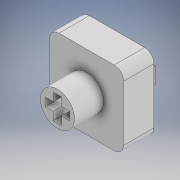
# Autodesk Inventor part: IPC MARK 7 key
Saved by Autodesk Inventor 2022 (Build 260153000, 153)
## iProperties
Created: 2021-12-31
Part Number: IPC MARK 7 key
Material: Generic
Document SubType Name: Modeling
Designer: solor
Density: 1 g/cm^3
Appearance: Default
Author: solor
Autodesk Inventor part; units mm, degrees
ref_plane "YZ Plane" through (0, 0, 0) normal (1, 0, 0) x (0, 1, 0)
ref_plane "XZ Plane" through (0, 0, 0) normal (0, 1, 0) x (-1, 0, 0)
sketch "Sketch1" plane through (0, 0, 0) normal (0, 0, 1) x (1, 0, 0)
  line L0 (14.6962, 12.74) -> (14.6962, 0) construction
  line L1 (10.61, 12.2) -> (1.53, 12.2)
  arc A0 (1.53, 12.2) -> (0, 10.67) centre (1.53, 10.67) ccw
  line L2 (0, 10.67) -> (0, 1.53)
  arc A1 (0, 1.53) -> (1.53, 0) centre (1.53, 1.53) ccw
  line L3 (1.53, 0) -> (10.61, 0)
  arc A2 (10.61, 0) -> (12.14, 1.53) centre (10.61, 1.53) ccw
  arc A3 (12.14, 10.67) -> (10.61, 12.2) centre (10.61, 10.67) ccw
  line L4 (12.14, 10.67) -> (12.14, 1.53)
  point P0 (0, 0)
  point P1 (0, 0)
  dimension "d10" = 12.74
  constraints: 10 end point, 8 point on circle, 4 centre point, 2 vertical, 1 point on line
  measures "d10" distance of L0.start L0.end
ref_plane "Work Plane1" through (0, 0, 5) normal (0, 0, 1) x (1, 0, 0)
sketch "Sketch2" plane through (0, 0, 5) normal (0, 0, 1) x (1, 0, 0)
  line L0 (10.88, 12.74) -> (1.8, 12.74) projected
  line L1 (10.88, 12.74) -> (1.8, 12.74) projected
  arc A0 (1.8, 12.74) -> (0, 10.94) centre (1.8, 10.94) ccw projected
  line L2 (0, 10.94) -> (0, 1.8) projected
  arc A1 (0, 1.8) -> (1.8, 0) centre (1.8, 1.8) ccw projected
  line L3 (1.8, 0) -> (10.88, 0) projected
  arc A2 (10.88, 0) -> (12.68, 1.8) centre (10.88, 1.8) ccw projected
  line L4 (12.68, 1.8) -> (12.68, 10.94) projected
  arc A3 (12.68, 10.94) -> (10.88, 12.74) centre (10.88, 10.94) ccw projected
  circle A4 centre (6.34, 6.37) radius 2.8
  line L5 (5.665, 8.395) -> (7.015, 8.395)
  line L6 (7.015, 4.345) -> (5.665, 4.345)
  line L7 (5.665, 4.345) -> (7.015, 8.395) construction
  line L8 (5.665, 8.395) -> (7.015, 4.345) construction
  line L9 (8.365, 5.695) -> (8.365, 7.045)
  line L10 (4.315, 7.045) -> (4.315, 5.695)
  line L11 (4.315, 5.695) -> (8.365, 7.045) construction
  line L12 (8.365, 5.695) -> (4.315, 7.045) construction
  line L13 (4.315, 5.695) -> (5.665, 5.695)
  line L14 (7.015, 5.695) -> (8.365, 5.695)
  line L15 (5.665, 4.345) -> (5.665, 5.695)
  line L16 (5.665, 7.045) -> (5.665, 8.395)
  line L17 (8.365, 7.045) -> (7.015, 7.045)
  line L18 (5.665, 7.045) -> (4.315, 7.045)
  line L19 (7.015, 8.395) -> (7.015, 7.045)
  line L20 (7.015, 5.695) -> (7.015, 4.345)
  point P0 (0, 0)
  dimension "d3" = 5.6
  dimension "d4" = 4.05
  dimension "d5" = 1.35
  dimension "d6" = 4.05
  dimension "d7" = 1.35
  constraints: 32 end point, 10 parallel, 8 perpendicular, 4 midpoint, 2 vertical, 1 centre point
  measures "d3" diameter of A4
  measures "d4" distance of L6.end L5.start
  measures "d5" distance of L5.start L5.end
  measures "d6" distance of L10.end L9.start
  measures "d7" distance of L9.end L9.start
extrude "Extrusion3" add sketch "Sketch1" along normal blind 5
sketch "Sketch3" plane through (0, 0, 5) normal (0, 0, 1) x (1, 0, 0)
  line L0 (10.61, 12.47) -> (1.53, 12.47)
  line L1 (10.61, 12.47) -> (1.53, 12.47)
  arc A0 (1.53, 12.47) -> (-0.27, 10.67) centre (1.53, 10.67) ccw
  line L2 (-0.27, 10.67) -> (-0.27, 1.53)
  arc A1 (-0.27, 1.53) -> (1.53, -0.27) centre (1.53, 1.53) ccw
  line L3 (1.53, -0.27) -> (10.61, -0.27)
  arc A2 (10.61, -0.27) -> (12.41, 1.53) centre (10.61, 1.53) ccw
  line L4 (12.41, 1.53) -> (12.41, 10.67)
  arc A3 (12.41, 10.67) -> (10.61, 12.47) centre (10.61, 10.67) ccw
  circle A4 centre (6.07, 6.1) radius 2.8
  line L5 (5.395, 8.125) -> (6.745, 8.125)
  line L6 (6.745, 4.075) -> (5.395, 4.075)
  line L7 (5.395, 4.075) -> (6.745, 8.125) construction
  line L8 (5.395, 8.125) -> (6.745, 4.075) construction
  line L9 (8.095, 5.425) -> (8.095, 6.775)
  line L10 (4.045, 6.775) -> (4.045, 5.425)
  line L11 (4.045, 5.425) -> (8.095, 6.775) construction
  line L12 (8.095, 5.425) -> (4.045, 6.775) construction
  line L13 (4.045, 5.425) -> (5.395, 5.425)
  line L14 (6.745, 5.425) -> (8.095, 5.425)
  line L15 (5.395, 4.075) -> (5.395, 5.425)
  line L16 (5.395, 6.775) -> (5.395, 8.125)
  line L17 (8.095, 6.775) -> (6.745, 6.775)
  line L18 (5.395, 6.775) -> (4.045, 6.775)
  line L19 (6.745, 8.125) -> (6.745, 6.775)
  line L20 (6.745, 5.425) -> (6.745, 4.075)
  line L21 (10.61, 12.2) -> (1.53, 12.2) projected
  line L22 (0, 10.67) -> (0, 1.53) projected
  point P0 (0, 0)
  point P1 (-0.27, -0.27)
  point P2 (6.07, 12.2)
  point P3 (0, 6.1)
  point P4 (6.07, 6.1)
  dimension "d14" = 5.6
  dimension "d15" = 4.05
  dimension "d16" = 1.35
  dimension "d17" = 4.05
  dimension "d18" = 1.35
  constraints: 42 end point, 10 parallel, 8 perpendicular, 8 point on circle, 6 midpoint, 5 centre point, 2 vertical
  measures "d14" diameter of A4
  measures "d15" distance of L6.end L5.start
  measures "d16" distance of L5.start L5.end
  measures "d17" distance of L10.end L9.start
  measures "d18" distance of L9.end L9.start
extrude "Extrusion4" add sketch "Sketch3" along normal blind 4.8 contours A4
sketch "Sketch4" plane through (0, 0, 0) normal (0, 0, -1) x (-1, 0, 0)
  line L0 (-13.9436, 0) -> (-13.9436, 2.266)
  line L1 (-15.5559, 0) -> (-15.5559, 6.84)
  line L2 (-1.53, 0) -> (-10.61, 0) projected
  line L3 (-11.7556, 9.6007) -> (-0.3844, 9.6007) construction
  line L4 (-0.3844, 9.6007) -> (-0.3844, 6.84) construction
  line L5 (-0.3844, 6.84) -> (-11.7556, 6.84) construction
  line L6 (-11.7556, 6.84) -> (-11.7556, 9.6007) construction
  line L7 (-7.4059, 5.316) -> (-4.7341, 5.316) construction
  line L8 (-4.7341, 5.316) -> (-4.7341, 2.266) construction
  line L9 (-4.7341, 2.266) -> (-7.4059, 2.266) construction
  line L10 (-7.4059, 2.266) -> (-7.4059, 5.316) construction
  line L11 (-8.7186, 6.9007) -> (-9.3925, 6.9007)
  line L12 (-9.3925, 6.9007) -> (-9.3925, 8.6905)
  line L13 (-9.3925, 8.6905) -> (-9.8826, 7.5352)
  line L14 (-9.8826, 7.5352) -> (-10.3465, 7.5352)
  line L15 (-10.3465, 7.5352) -> (-10.8366, 8.6905)
  line L16 (-10.8366, 8.6905) -> (-10.8366, 6.9007)
  line L17 (-10.8366, 6.9007) -> (-11.4755, 6.9007)
  line L18 (-11.4755, 6.9007) -> (-11.4755, 9.6007)
  line L19 (-11.4755, 9.6007) -> (-10.6944, 9.6007)
  line L20 (-10.6944, 9.6007) -> (-10.0949, 8.2682)
  line L21 (-10.0949, 8.2682) -> (-9.4997, 9.6007)
  line L22 (-9.4997, 9.6007) -> (-8.7186, 9.6007)
  line L23 (-8.7186, 9.6007) -> (-8.7186, 6.9007)
  line L24 (-8.4495, 6.9007) -> (-7.5371, 9.6007)
  line L25 (-7.5371, 9.6007) -> (-6.7976, 9.6007)
  line L26 (-6.7976, 9.6007) -> (-5.8852, 6.9007)
  line L27 (-5.8852, 6.9007) -> (-6.5831, 6.9007)
  line L28 (-6.5831, 6.9007) -> (-6.7516, 7.4521)
  line L29 (-6.7516, 7.4521) -> (-7.6006, 7.4521)
  line L30 (-7.6006, 7.4521) -> (-7.7712, 6.9007)
  line L31 (-7.7712, 6.9007) -> (-8.4495, 6.9007)
  line L32 (-6.9004, 7.9422) -> (-7.1761, 8.8349)
  line L33 (-7.1761, 8.8349) -> (-7.454, 7.9422)
  line L34 (-7.454, 7.9422) -> (-6.9004, 7.9422)
  line L35 (-3.1217, 6.9007) -> (-3.9466, 6.9007)
  line L36 (-3.9466, 6.9007) -> (-4.6971, 7.8919)
  line L37 (-4.6971, 7.8919) -> (-4.9421, 7.8919)
  line L38 (-4.9421, 7.8919) -> (-4.9421, 6.9007)
  line L39 (-4.9421, 6.9007) -> (-5.616, 6.9007)
  line L40 (-5.616, 6.9007) -> (-5.616, 9.6007)
  line L41 (-5.616, 9.6007) -> (-4.5308, 9.6007)
  spline S0 degree 2 poles (-4.5308, 9.6007) (-4.3054, 9.6007) (-3.9728, 9.5438) (-3.8306, 9.4563) knots 0 0 0 1 2 2 2
  spline S1 degree 2 poles (-3.8306, 9.4563) (-3.6862, 9.3644) (-3.5155, 9.0778) (-3.5155, 8.859) knots 0 0 0 1 2 2 2
  spline S2 degree 2 poles (-3.5155, 8.859) (-3.5155, 8.5505) (-3.7956, 8.1632) (-4.0297, 8.0494) knots 0 0 0 1 2 2 2
  line L42 (-4.0297, 8.0494) -> (-3.1217, 6.9007)
  spline S3 degree 2 poles (-4.2113, 8.7736) (-4.2113, 8.8765) (-4.2901, 9.0231) (-4.3798, 9.0625) knots 0 0 0 1 2 2 2
  spline S4 degree 2 poles (-4.3798, 9.0625) (-4.4433, 9.0887) (-4.5986, 9.104) (-4.7146, 9.104) knots 0 0 0 1 2 2 2
  line L43 (-4.7146, 9.104) -> (-4.9421, 9.104)
  line L44 (-4.9421, 9.104) -> (-4.9421, 8.3776)
  line L45 (-4.9421, 8.3776) -> (-4.7474, 8.3776)
  spline S5 degree 2 poles (-4.7474, 8.3776) (-4.6074, 8.3776) (-4.4082, 8.4126) (-4.3404, 8.4673) knots 0 0 0 1 2 2 2
  spline S6 degree 2 poles (-4.3404, 8.4673) (-4.2748, 8.5198) (-4.2113, 8.6599) (-4.2113, 8.7736) knots 0 0 0 1 2 2 2
  line L46 (-0.5552, 6.9007) -> (-1.3757, 6.9007)
  line L47 (-1.3757, 6.9007) -> (-2.1087, 7.9969)
  line L48 (-2.1087, 7.9969) -> (-2.2421, 7.8131)
  line L49 (-2.2421, 7.8131) -> (-2.2421, 6.9007)
  line L50 (-2.2421, 6.9007) -> (-2.9204, 6.9007)
  line L51 (-2.9204, 6.9007) -> (-2.9204, 9.6007)
  line L52 (-2.9204, 9.6007) -> (-2.2421, 9.6007)
  line L53 (-2.2421, 9.6007) -> (-2.2421, 8.3951)
  line L54 (-2.2421, 8.3951) -> (-1.3757, 9.6007)
  line L55 (-1.3757, 9.6007) -> (-0.5946, 9.6007)
  line L56 (-0.5946, 9.6007) -> (-1.5573, 8.347)
  line L57 (-1.5573, 8.347) -> (-0.5552, 6.9007)
  line L58 (-4.9219, 4.7104) -> (-6.2245, 2.266)
  line L59 (-6.2245, 2.266) -> (-7.0747, 2.266)
  line L60 (-7.0747, 2.266) -> (-5.7128, 4.7401)
  line L61 (-5.7128, 4.7401) -> (-7.1662, 4.7401)
  line L62 (-7.1662, 4.7401) -> (-7.1662, 5.316)
  line L63 (-7.1662, 5.316) -> (-4.9219, 5.316)
  line L64 (-4.9219, 5.316) -> (-4.9219, 4.7104)
  point P0 (0, 0)
  point P1 (-6.07, 0)
  point P2 (-6.07, 2.266)
  point P3 (-6.07, 6.84)
  point P4 (-6.07, 2.266)
  dimension "d21" = 2.266
  dimension "d22" = 6.84
  constraints: 4 end point, 3 midpoint, 2 vertical, 4 other
  measures "d21" distance of L0.start L0.end
  measures "d22" distance of L1.start L1.end
extrude "Extrusion5" add sketch "Sketch4" along normal blind 0.9
body "Solid2"
